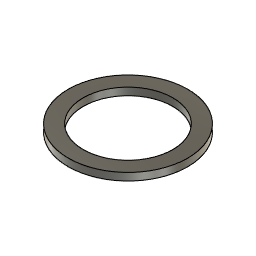
IR Sensor Shield and Bearing (Autodesk Fusion 360 design; units mm, degrees)
Autodesk Fusion 360 part; units mm, degrees
cylinder "CylinderPrimitive1" add diameter 19.05 height 1.1906 placed x (1, 0, 0) y (0, 1, 0) z (0, 0, 1) at (0, 0, 0)
hole "Hole1" at (0, 0, 1.1906) direction (0, 0, -1) diameter 14.3002 depth 7.62 tip angle 180
equation "d1 = ( 0.75 / 16 ) * 1 in"
